# Autodesk Inventor part: Roller Chain
Saved by Autodesk Inventor 2016 (Build 200138000, 138)
## iProperties
Created: 2016-01-17
Part Number: Roller Chain
Material: Generic
Document SubType Name: Modeling
Designer: gus
Mass: 37.3283 g
Surface Area: 238.562 cm^2
Volume: 37.3283 cm^3
Density: 1 g/cm^3
Appearance: Clear - Blue
CustomPartVersion: 1
Author: gus
Autodesk Inventor part; units mm, degrees
ref_plane "Work Plane2" through (92.3994, 87.8892, 0) normal (-1, 0, 0) x (0, 0, 1)
ref_plane "Work Plane3" through (0, 0, 0) normal (0.6338453, 0.7734598, 0) x (0, 0, 1)
sketch "Path" plane through (0, 0, 0) normal (0, 0, 1) x (1, 0, 0)
  arc A0 (108.7359, 76.5248) -> (81.8661, 104.7735) centre (92.3994, 87.8892) ccw
  arc A1 (-24.1158, 38.6562) -> (37.402, -26.0186) centre (0, 0) ccw
  line L0 (-24.1158, 38.6562) -> (81.8661, 104.7735)
  line L1 (108.7359, 76.5248) -> (37.402, -26.0186)
  dimension "d31" = 8.9916
  constraints: 4 end point, 4 point on circle, 2 centre point
ref_plane "Section Plane" through (81.8661, 104.7735, 0) normal (-0.8484349, -0.5292998, 0) x (0, 0, 1)
sketch "Section Sketch" plane through (81.8661, 104.7735, 0) normal (-0.8484349, -0.5292998, 0) x (0, 0, 1)
  line L0 (-6.35, -1.7907) -> (6.35, -1.7907)
  line L1 (6.35, -1.7907) -> (6.35, 1.7907)
  line L2 (6.35, 1.7907) -> (-6.35, 1.7907)
  line L3 (-6.35, 1.7907) -> (-6.35, -1.7907)
  line L4 (-2.3876, -2.54) -> (2.3876, -2.54)
  line L5 (2.3876, -2.54) -> (2.3876, 2.54)
  line L6 (2.3876, 2.54) -> (-2.3876, 2.54)
  line L7 (-2.3876, 2.54) -> (-2.3876, -2.54)
  line L8 (-2.3876, 0) -> (2.3876, 0) construction
  line L9 (-4.9276, -4.4958) -> (-2.3876, -4.4958)
  line L10 (-2.3876, -4.4958) -> (-2.3876, 4.4958)
  line L11 (-2.3876, 4.4958) -> (-4.9276, 4.4958)
  line L12 (-4.9276, 4.4958) -> (-4.9276, -4.4958)
  line L13 (2.3876, -4.4958) -> (4.9276, -4.4958)
  line L14 (4.9276, -4.4958) -> (4.9276, 4.4958)
  line L15 (4.9276, 4.4958) -> (2.3876, 4.4958)
  line L16 (2.3876, 4.4958) -> (2.3876, -4.4958)
  line L17 (-6.35, 0) -> (6.35, 0) construction
  point P0 (0, 0)
  point P1 (0, 0)
  dimension "d21" = 3.5814
  dimension "d22" = 5.08
  dimension "d23" = 4.7752
  dimension "d24" = 2.54
  dimension "d31" = 8.9916
  dimension "d32" = 12.7
  constraints: 36 end point, 8 midpoint, 8 parallel, 4 horizontal, 4 perpendicular, 3 collinear, 1 coincident, 1 other
  measures "d21" distance between parallel lines of L2 L0
  measures "d22" distance between parallel lines of L6 L4
  measures "d23" distance between parallel lines of L5 L7
  measures "d24" distance between parallel lines of L12 L10
  measures "d31" distance between parallel lines of L11 L9
  measures "d32" distance between parallel lines of L1 L3
sweep "Solid" add profiles "Section Sketch" path "Path"
pattern_of_one "Strand Pattern"
equation "\"d21\" = da_d2"
equation "\"d22\" = da_d1"
equation "\"d23\" = da_b1"
equation "\"d24\" = da_t1 + da_t2"
equation "\"d30\" = da_pt"
equation "\"da_p\" = 9.525"
equation "\"da_b1\" = 4.7752"
equation "\"da_h2\" = 8.9916"
equation "\"da_h3\" = 7.7978"
equation "\"da_d1\" = 5.08"
equation "\"da_d2\" = 3.5814"
equation "\"da_pt\" = 10.1346"
equation "\"da_b\" = 12.7"
equation "\"da_t1\" = 1.27"
equation "\"da_t2\" = 1.27"
body "Solid1"
